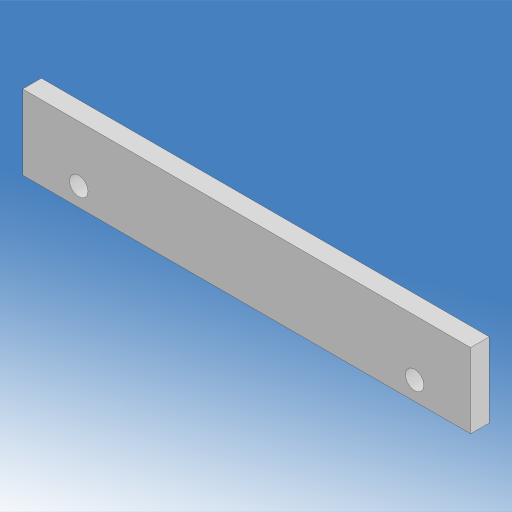
# Autodesk Inventor part: Testblock
Saved by Autodesk Inventor 2024 (Build 280153000, 153)
## iProperties
Created: 2024-03-30
Part Number: Testblock
Material: Generic
Document SubType Name: Modeling
Designer: seene
Density: 1 g/cm^3
Appearance: Default
Author: seene
Autodesk Inventor part; units mm, degrees
ref_plane "YZ Plane" through (0, 0, 0) normal (1, 0, 0) x (0, 1, 0)
ref_plane "XZ Plane" through (0, 0, 0) normal (0, 1, 0) x (-1, 0, 0)
ref_plane "XY Plane" through (0, 0, 0) normal (0, 0, 1) x (1, 0, 0)
sketch "Sketch1" plane through (0, 0, 0) normal (0, 0, 1) x (1, 0, 0)
  line L0 (0, 0) -> (609.6, 0)
  line L1 (609.6, 0) -> (609.6, 101.6)
  line L2 (609.6, 101.6) -> (0, 101.6)
  line L3 (0, 101.6) -> (0, 0)
  circle A0 centre (76.2, 25.4) radius 12.7
  circle A1 centre (533.4, 25.4) radius 12.7
  dimension "d0" = 609.6
  dimension "d1" = 101.6
  dimension "d2" = 25.4
  dimension "d3" = 25.4
  dimension "d4" = 76.2
  dimension "d5" = 76.2
  dimension "d6" = 25.4
  constraints: 8 end point, 2 centre point, 2 parallel, 1 horizontal, 1 horizontal alignment, 1 perpendicular
  measures "d0" distance of L1.end L2.end
  measures "d1" distance of L2.end L0.start
  measures "d2" diameter of A0
  measures "d3" diameter of A1
  measures "d4" distance from line of A0.centre L3
  measures "d5" distance from line of L1 A1.centre
  measures "d6" distance from line of A0.centre L0
extrude "Extrusion1" add sketch "Sketch1" along normal blind 25.4
body "Solid1"
